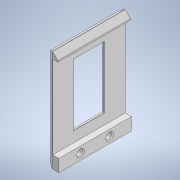
# Autodesk Inventor part: Скоба
Saved by Autodesk Inventor 2021 (Build 250183000, 183)
## iProperties
Created: 2024-05-10
Part Number: Скоба
Material: Типовые
Document SubType Name: Modeling
Designer: Мария
Density: 1 g/cm^3
Appearance: По умолчанию
Author: Мария
Autodesk Inventor part; units mm, degrees
ref_plane "YZ Plane" through (0, 0, 0) normal (1, 0, 0) x (0, 1, 0)
ref_plane "XZ Plane" through (0, 0, 0) normal (0, 1, 0) x (-1, 0, 0)
ref_plane "XY Plane" through (0, 0, 0) normal (0, 0, 1) x (1, 0, 0)
sketch "Эскиз1" plane through (0, 0, 0) normal (0, 0, 1) x (1, 0, 0)
  line L0 (0, 0) -> (0, 49.2)
  line L1 (0, 49.2) -> (4.5, 49.2)
  line L2 (4.5, 49.2) -> (4.5, 46)
  line L3 (4.5, 46) -> (2, 46)
  line L4 (2, 46) -> (2, 6)
  line L5 (2, 6) -> (5, 6)
  line L6 (5, 6) -> (5, 0)
  line L7 (5, 0) -> (0, 0)
  dimension "d1" = 3
  dimension "d2" = 2.5
  dimension "d3" = 2
  dimension "d4" = 6
  dimension "d6" = 3.2
  dimension "d17" = 40
  constraints: 16 end point, 2 parallel, 1 horizontal, 1 perpendicular, 1 vertical
  measures "d1" distance of L4.end L5.end
  measures "d2" distance of L2.end L3.end
  measures "d3" distance between parallel lines of L0 L4
  measures "d4" distance between parallel lines of L7 L5
  measures "d6" distance between parallel lines of L1 L3
  measures "d17" distance from line of L2.end L5
extrude "Выдавливание1" add sketch "Эскиз1" along normal blind 35
sketch "Эскиз2" plane through (5, 0, 0) normal (1, 0, 0) x (0, 0, -1)
  circle A0 centre (-24.5, 3) radius 1.4
  circle A1 centre (-10.5, 3) radius 1.4
  line L0 (0, 0) -> (-35, 0) projected
  line L1 (0, 0) -> (-35, 0) projected
  line L2 (0, 6) -> (-35, 6) projected
  point P0 (-17.5, 0)
  dimension "d9" = 2.8
  dimension "d10" = 2.8
  dimension "d11" = 14
  dimension "d12" = 7
  dimension "d13" = 3
  dimension "d14" = 6
  constraints: 2 centre point, 1 horizontal alignment, 1 midpoint
  measures "d9" diameter of A0
  measures "d10" diameter of A1
  measures "d11" distance of A1.centre A0.centre
  measures "d12" horizontal distance of A0.centre point (-17.5, 0)
  measures "d13" distance from line of L0 A0.centre
  measures "d14" distance between parallel lines of L2 L0
extrude "Выдавливание2" cut sketch "Эскиз2" against normal blind 4.6
chamfer "Фаска1" distance 2.5 angle 45 1 edges at (4.5, 49.2, 17.5) measured on face at (4.5, 47.0667, 11.6667)
chamfer "Фаска2" distance 1 angle 60 4 edges at (0, 0, 17.5) (0, 49.2, 17.5) (0, 24.6, 0) (0, 24.6, 35) measured on face at (0, 32.8, 11.6667)
sketch "Эскиз3" plane through (2, 6, 0) normal (1, 0, 0) x (0, 0, -1)
  line L0 (-25, 5) -> (-10, 5)
  line L1 (-10, 5) -> (-10, 35)
  line L2 (-10, 35) -> (-25, 35)
  line L3 (-25, 35) -> (-25, 5)
  line L4 (-35, 0) -> (-35, 40) projected
  line L5 (0, 0) -> (0, 40) projected
  line L6 (0, 40) -> (-35, 40) projected
  point P0 (0, -6)
  dimension "d24" = 15
  dimension "d25" = 30
  dimension "d26" = 40
  dimension "d27" = 35
  dimension "d28" = 10
  dimension "d29" = 5
  constraints: 8 end point, 2 parallel, 1 horizontal, 1 perpendicular
  measures "d24" distance between parallel lines of L1 L3
  measures "d25" distance between parallel lines of L0 L2
  measures "d26" distance of L4.end L4.start
  measures "d27" distance between parallel lines of L5 L4
  measures "d28" distance between parallel lines of L4 L3
  measures "d29" distance between parallel lines of L6 L2
extrude "Выдавливание3" cut sketch "Эскиз3" against normal through all
chamfer "Фаска3" distance 0.5 angle 45 2 edges at (5, 3, 25.9) (5, 3, 11.9)
chamfer "Фаска4" distance 1 angle 60 4 edges at (0, 26, 10) (0, 11, 17.5) (0, 41, 17.5) (0, 26, 25) measured on face at (0, 20.0667, 31)
equation "\"d13\" = 0.5 * d14"
equation "\"d28\" = -0.5 * d24 + 0.5 * d27"
equation "\"d29\" = -0.5 * d25 + 0.5 * d26"
